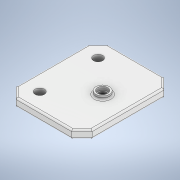
# Autodesk Inventor part: base1
Saved by Autodesk Inventor 2022 (Build 260153000, 153)
## iProperties
Created: 2022-06-14
Part Number: base1
Material: ABS プラスチック
Document SubType Name: Modeling
Designer: yuto6
Density: 1.06 g/cm^3
Appearance: 滑らか - 白
Author: yuto6
Autodesk Inventor part; units mm, degrees
ref_plane "YZ Plane" through (0, 0, 0) normal (1, 0, 0) x (0, 1, 0)
ref_plane "XZ Plane" through (0, 0, 0) normal (0, 1, 0) x (-1, 0, 0)
ref_plane "XY Plane" through (0, 0, 0) normal (0, 0, 1) x (1, 0, 0)
sketch "スケッチ1" plane through (0, 0, 0) normal (0, 1, 0) x (-1, 0, 0)
  line L0 (22.5, -27.3) -> (-22.5, -27.3)
  line L1 (-22.5, -27.3) -> (-22.5, 27.3)
  line L2 (-22.5, 27.3) -> (22.5, 27.3)
  line L3 (22.5, 27.3) -> (22.5, -27.3)
  line L4 (22.5, -27.3) -> (-22.5, 27.3) construction
  line L5 (-22.5, -27.3) -> (22.5, 27.3) construction
  point P0 (0, 0)
  dimension "d0" = 45
  dimension "d1" = 54.6
  constraints: 12 end point, 2 midpoint, 2 parallel, 1 horizontal, 1 perpendicular
  measures "d0" distance of L1.end L2.end
  measures "d1" distance of L2.end L0.start
extrude "押し出し1" add sketch "スケッチ1" along normal blind 5
sketch "スケッチ2" plane through (0, 5, 0) normal (0, 1, 0) x (1, 0, 0)
  line L0 (-22.5, 27.3) -> (-22.5, -27.3) projected
  line L1 (-22.5, -27.3) -> (22.5, -27.3) projected
  line L2 (22.5, 27.3) -> (-22.5, 27.3) projected
  point P0 (0, 0)
  point P1 (-12.5, -17.3)
  point P2 (-12.5, 17.3)
  dimension "d4" = 10
  dimension "d5" = 10
  dimension "d6" = 10
  constraints: 1 vertical alignment
  measures "d4" distance from line of L0 point (-12.5, -17.3)
  measures "d5" distance from line of L1 point (-12.5, -17.3)
  measures "d6" distance from line of L2 point (-12.5, 17.3)
hole "穴1" at (-12.5, 5, 17.3) at (-12.5, 5, -17.3) direction (0, -1, 0) diameter 5.5 end through all clearance for "Flat Head Machine Screw" size "M5" standard "Ansi Metric M Profile"
chamfer "面取り1" distance 6 angle 45 4 edges at (22.5, 2.5, -27.3) (22.5, 2.5, 27.3) (-22.5, 2.5, -27.3) (-22.5, 2.5, 27.3)
sketch "スケッチ5" plane through (0, 5, 0) normal (0, 1, 0) x (1, 0, 0)
  circle A0 centre (-12.5, -17.3) radius 2.75 projected
  point P0 (0, 0)
  point P1 (7.5, 0)
  dimension "d43" = 20
  constraints: 1 horizontal alignment
  measures "d43" horizontal distance of A0.centre point (7.5, 0)
hole "穴2" at (7.5, 5, 0) direction (0, -1, 0) diameter 4.3 end through all clearance for "Flat Head Machine Screw" size "M4" standard "Ansi Metric M Profile"
sketch "スケッチ6" plane through (0, 5, 0) normal (0, 1, 0) x (1, 0, 0)
  circle A0 centre (7.5, 0) radius 2.15 projected
  circle A1 centre (7.5, 0) radius 3
  circle A2 centre (7.5, 0) radius 4
  point P0 (0, 0)
  dimension "d51" = 6
  dimension "d52" = 8
  constraints: 2 centre point, 2 coincident
  measures "d51" diameter of A1
  measures "d52" diameter of A2
extrude "押し出し4" add sketch "スケッチ6" along normal blind 2 contours A2
fillet "フィレット1" radius 1 1 edges at (3.5, 5, 0)
sketch "スケッチ7" plane through (0, 0, 0) normal (0, -1, 0) x (1, 0, 0)
  circle A0 centre (7.5, 0) radius 2.15 projected
  line L0 (7.5, -4.3301) -> (3.75, -2.1651)
  line L1 (3.75, -2.1651) -> (3.75, 2.1651)
  line L2 (3.75, 2.1651) -> (7.5, 4.3301)
  line L3 (7.5, 4.3301) -> (11.25, 2.1651)
  line L4 (11.25, 2.1651) -> (11.25, -2.1651)
  line L5 (11.25, -2.1651) -> (7.5, -4.3301)
  point P0 (0, 0)
  dimension "d56" = 7.5
  constraints: 12 end point, 1 coincident, 13 other
  measures "d56" distance between parallel lines of L4 L1
extrude "押し出し5" cut sketch "スケッチ7" against normal blind 2
fillet "フィレット2" radius 1 16 edges at (-22.5, 5, 0) (-19.5, 5, 24.3) (0, 5, 27.3) (19.5, 5, 24.3) (22.5, 5, 0) (19.5, 5, -24.3) (0, 5, -27.3) (-19.5, 5, -24.3) (0, 0, -27.3) (-19.5, 0, -24.3) (19.5, 0, -24.3) (22.5, 0, 0) (19.5, 0, 24.3) (0, 0, 27.3) (-19.5, 0, 24.3) (-22.5, 0, 0)
equation "\"d6\" = d5"
